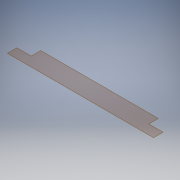
# Autodesk Inventor part: Tampa Gaveta
Saved by Autodesk Inventor 2018 (Build 220112000, 112)
## iProperties
Created: 2018-07-08
Part Number: Tampa Gaveta
Material: PMMA plástico
Document SubType Name: Chapa de metal
Designer: Regner
Density: 1.188 g/cm^3
Sheet Metal Rule: Padrão_mm
Appearance: Policarbonato - Fumê
Author: Regner
Autodesk Inventor part; units mm, degrees
ref_plane "YZ Plane" through (0, 0, 0) normal (1, 0, 0) x (0, 1, 0)
ref_plane "XZ Plane" through (0, 0, 0) normal (0, 1, 0) x (-1, 0, 0)
ref_plane "XY Plane" through (0, 0, 0) normal (0, 0, 1) x (1, 0, 0)
sketch "Esboço1" plane through (0, 0, 0) normal (0, 0, 1) x (1, 0, 0)
  line L0 (123.4, -20) -> (-123.4, -20)
  line L1 (-123.4, -20) -> (-123.4, 20)
  line L2 (-123.4, 20) -> (123.4, 20)
  line L3 (123.4, 20) -> (123.4, -20)
  line L4 (123.4, -20) -> (-123.4, 20) construction
  line L5 (-123.4, -20) -> (123.4, 20) construction
  line L6 (-123.4, -20) -> (-153.4, -20)
  line L7 (-153.4, -20) -> (-153.4, 0)
  line L8 (-153.4, 0) -> (-123.4, 0)
  line L9 (-123.4, 0) -> (-123.4, -20)
  line L10 (123.4, -20) -> (153.4, -20)
  line L11 (153.4, -20) -> (153.4, 0)
  line L12 (153.4, 0) -> (123.4, 0)
  line L13 (123.4, 0) -> (123.4, -20)
  point P0 (0, 0)
  dimension "d0" = 246.8
  dimension "d1" = 40
  dimension "d2" = 30
  dimension "d3" = 20
  dimension "d4" = 30
  dimension "d5" = 20
  measures "d0" distance of L1.end L2.end
  measures "d1" distance of L0.end L1.end
  measures "d2" distance of L7.end L8.end
  measures "d3" distance of L6.end L7.end
  measures "d4" distance of L12.end L11.end
  measures "d5" distance of L11.end L10.end
extrude "Placa1" add sketch "Esboço1" along normal blind 0.5
equation "\"d6\" = Espessura"
equation "\"Raio_vergadura\" = Espessura"
equation "\"Largura_alívio_de_vergadura\" = Espessura"
equation "\"Profundidade_alívio_de_vergadura\" = 0.5 * Espessura"
equation "\"Tamanho_alívio_de_dobra\" = 4 * Espessura"
equation "\"Remanescente_mínimo\" = 2 * Espessura"
equation "\"Raiodetransição\" = Raio_vergadura"
equation "\"Tamanho_de_raio_de_Jacobi\" = Raio_vergadura"
equation "\"TamanhoFolga\" = Espessura"
equation "\"Espessura\" = 0.5"
